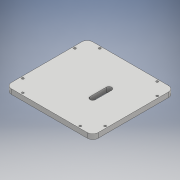
# Autodesk Inventor part: Parte6
Saved by Autodesk Inventor 2017 (Build 210142000, 142)
## iProperties
Part Number: Parte6
Material: Generico
Document SubType Name: Modeling
Designer: Federico
Density: 1 g/cm^3
Appearance: Default
Author: Federico
Autodesk Inventor part; units mm, degrees
ref_plane "YZ Plane" through (0, 0, 0) normal (1, 0, 0) x (0, 1, 0)
ref_plane "XZ Plane" through (0, 0, 0) normal (0, 1, 0) x (-1, 0, 0)
ref_plane "XY Plane" through (0, 0, 0) normal (0, 0, 1) x (1, 0, 0)
sketch "Schizzo1" plane through (0, 0, 0) normal (0, 0, 1) x (1, 0, 0)
  line L0 (75, -65) -> (75, 65)
  line L1 (65, 75) -> (-75, 75)
  line L2 (-85, 65) -> (-85, -65)
  line L3 (-75, -75) -> (65, -75)
  arc A0 (-85, -65) -> (-75, -75) centre (-75, -65) ccw
  arc A1 (-75, 75) -> (-85, 65) centre (-75, 65) ccw
  arc A2 (75, 65) -> (65, 75) centre (65, 65) ccw
  arc A3 (65, -75) -> (75, -65) centre (65, -65) ccw
  circle A4 centre (-81, 48) radius 2
  circle A5 centre (-81, -48) radius 2
  circle A6 centre (71, 48) radius 2
  circle A7 centre (71, -48) radius 2
  circle A8 centre (-58, -71) radius 2
  circle A9 centre (-58, 71) radius 2
  circle A10 centre (48, 71) radius 2
  circle A11 centre (48, -71) radius 2
  dimension "d32" = 10
  dimension "d42" = 4
  dimension "d43" = 4
  dimension "d45" = 4
  dimension "d46" = 4
  dimension "d53" = 4
  dimension "d54" = 4
  dimension "d55" = 4
  dimension "d56" = 4
  constraints: 12 centre point, 8 end point, 8 point on circle, 8 tangent, 3 equal radius, 1 perpendicular
  measures "d32" radius of A0
  measures "d42" diameter of A4
  measures "d43" diameter of A5
  measures "d45" diameter of A6
  measures "d46" diameter of A7
  measures "d53" diameter of A8
  measures "d54" diameter of A9
  measures "d55" diameter of A10
  measures "d56" diameter of A11
extrude "Estrusione2" add sketch "Schizzo1" along normal blind 9
sketch "Schizzo2" plane through (0, 0, 0) normal (0, 0, -1) x (-1, 0, 0)
  line L0 (75, -65) -> (75, 65)
  line L1 (65, 75) -> (-75, 75)
  line L2 (-85, 65) -> (-85, -65)
  line L3 (-75, -75) -> (65, -75)
  circle A0 centre (0, -36) radius 2
  circle A1 centre (0, 36) radius 2
  circle A2 centre (55, -36) radius 2
  circle A3 centre (55, 36) radius 2
  circle A4 centre (-75, -36) radius 2
  circle A5 centre (-75, 36) radius 2
  arc A6 (-85, -65) -> (-75, -75) centre (-75, -65) ccw
  arc A7 (-75, 75) -> (-85, 65) centre (-75, 65) ccw
  arc A8 (75, 65) -> (65, 75) centre (65, 65) ccw
  arc A9 (65, -75) -> (75, -65) centre (65, -65) ccw
  line L4 (-25, -20) -> (-25, -20)
  line L5 (-20, -15) -> (-20, 15)
  line L6 (-25, 20) -> (-25, 20)
  line L7 (-30, 15) -> (-30, -15)
  arc A10 (-30, -15) -> (-25, -20) centre (-25, -15) ccw
  arc A11 (-25, -20) -> (-20, -15) centre (-25, -15) ccw
  arc A12 (-20, 15) -> (-25, 20) centre (-25, 15) ccw
  arc A13 (-25, 20) -> (-30, 15) centre (-25, 15) ccw
  point P0 (0, 0)
  point P1 (0, 0)
  point P2 (-25, 0)
  dimension "d64" = 4
  dimension "d65" = 4
  dimension "d66" = 4
  dimension "d67" = 4
  dimension "d68" = 4
  dimension "d69" = 4
  dimension "d70" = 10
  dimension "d71" = 5
  constraints: 16 end point, 16 point on circle, 16 tangent, 14 centre point, 6 equal radius, 2 parallel, 2 perpendicular, 1 horizontal
  measures "d64" diameter of A0
  measures "d65" diameter of A1
  measures "d66" diameter of A2
  measures "d67" diameter of A3
  measures "d68" diameter of A4
  measures "d69" diameter of A5
  measures "d70" radius of A6
  measures "d71" radius of A10
move or copy body "Sposta corpo1" bodies to move or copy 1 copy no translate (10, 0, 0)
extrude "Estrusione3" cut sketch "Schizzo2" against normal blind 9 contours A11 A10 L7 A13 A12 L5
